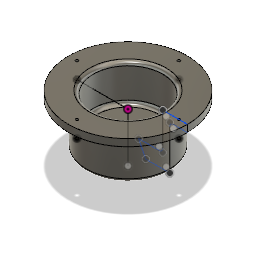
_distance sensing base.b2dd820b-1519-46c9-ab9c-6e6810837444 (Autodesk Fusion 360 design; units mm, degrees)
Autodesk Fusion 360 part; units mm, degrees
note: some values were not read from the file. Set by a fixed rule: which sketch regions a step uses.
sketch "Sketch1" plane through (0, 0, 0) normal (0, 0, 1) x (1, 0, 0)
  line L0 (0, 0) -> (0, -69.4878)
  line L1 (15, -28.6078) -> (25, -48.6078)
  line L2 (15, -28.6078) -> (44, -28.6078)
  line L3 (25, -48.6078) -> (54, -48.6078)
  line L4 (49, -23.6078) -> (49, 18.2922)
  line L5 (59, -43.6078) -> (59, 8.2922)
  line L6 (54, 23.2922) -> (84, 23.2922)
  line L7 (64, 13.2922) -> (84, 13.2922)
  line L8 (84, 23.2922) -> (84, 13.2922)
  arc A0 (44, -28.6078) -> (49, -23.6078) centre (44, -23.6078) ccw
  arc A1 (54, -48.6078) -> (59, -43.6078) centre (54, -43.6078) ccw
  arc A2 (64, 13.2922) -> (59, 8.2922) centre (64, 8.2922) ccw
  arc A3 (54, 23.2922) -> (49, 18.2922) centre (54, 18.2922) ccw
  point P0 (15, -28.6078)
  point P1 (25, -48.6078)
  point P2 (49, -28.6078)
  point P3 (59, -48.6078)
  point P4 (49, 23.2922)
  point P5 (59, 13.2922)
  dimension "d2" = 15
  dimension "d4" = 25
  dimension "d19" = 34
  dimension "d20" = 34
  dimension "d21" = 51.9
  dimension "d22" = 61.9
  dimension "d23" = 35
  dimension "d25" = 5
  measures "d2" distance of L0 P0
  measures "d4" distance of L0 P1
  measures "d19" distance of P0 P2
  measures "d20" distance of P1 P3
  measures "d21" distance of P2 P4
  measures "d22" distance of P3 P5
  measures "d23" distance of P4 L6.end
  measures "d25" radius of A0
revolve "Revolve1" add sketch "Sketch1" angle 360 about axis through (0, 0, 0) along (0, -1, 0)
sketch "Sketch2" plane through (0, 0, 0) normal (0, 1, 0) x (1, 0, 0)
  circle A0 centre (-72, 0) radius 1.95
  line L0 (-72, 0) -> (0, 0)
  circle A1 centre (0, -72) radius 1.95
  circle A2 centre (72, 0) radius 1.95
  circle A3 centre (0, 72) radius 1.95
  dimension "d13" = 3.9
  dimension "d14" = 72
  dimension "d16" = 360
  measures "d13" diameter of A0
  measures "d14" distance of A0.centre L0.end
extrude "Extrude1" cut sketch "Sketch2" along normal mid plane 200
